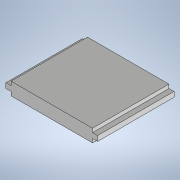
# Autodesk Inventor part: Крышка аккумулятора
Saved by Autodesk Inventor 2020 (Build 240168000, 168)
## iProperties
Created: 2021-04-26
Part Number: Крышка аккумулятора
Material: Типовые
Document SubType Name: Modeling
Designer: Антон
Density: 1 g/cm^3
Appearance: По умолчанию
Author: Антон
Autodesk Inventor part; units mm, degrees
ref_plane "YZ Plane" through (0, 0, 0) normal (1, 0, 0) x (0, 1, 0)
ref_plane "XZ Plane" through (0, 0, 0) normal (0, 1, 0) x (-1, 0, 0)
ref_plane "XY Plane" through (0, 0, 0) normal (0, 0, 1) x (1, 0, 0)
sketch "Эскиз1" plane through (0, 0, 0) normal (0, 0, 1) x (1, 0, 0)
  line L0 (0, 0) -> (32, 0)
  line L1 (32, 0) -> (32, 5)
  line L2 (32, 5) -> (0, 5)
  line L3 (0, 5) -> (0, 0)
  line L4 (32, 3.5) -> (34, 3.5)
  line L5 (34, 3.5) -> (34, 1.5)
  line L6 (34, 1.5) -> (32, 1.5)
  line L7 (32, 1.5) -> (32, 3.5)
  line L8 (-2, 1.5) -> (0, 1.5)
  line L9 (0, 1.5) -> (0, 3.5)
  line L10 (0, 3.5) -> (-2, 3.5)
  line L11 (-2, 3.5) -> (-2, 1.5)
  point P0 (32, 2.5)
  point P1 (0, 2.5)
  dimension "d32" = 32
  dimension "d33" = 5
  dimension "d34" = 2
  dimension "d35" = 2
  constraints: 24 end point, 6 parallel, 4 midpoint, 3 horizontal, 3 perpendicular, 2 equal length
  measures "d32" distance of L2.end L1.end
  measures "d33" distance of L1.end L0.end
  measures "d34" distance of L5.end L6.end
  measures "d35" distance of L4.end L5.end
extrude "Выдавливание1" add sketch "Эскиз1" along normal blind 30
